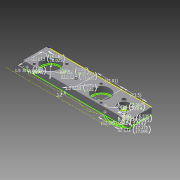
# Autodesk Inventor part: mount
Saved by Autodesk Inventor 2014 (Build 180170000, 170)
## iProperties
Created: 2013-09-13
Part Number: mount
Material: Generic
Document SubType Name: Modeling
Designer: Brandon
Density: 1 g/cm^3
Appearance: Default
Author: Brandon
Autodesk Inventor part; units mm, degrees
ref_plane "YZ Plane" through (0, 0, 0) normal (1, 0, 0) x (0, 1, 0)
ref_plane "XZ Plane" through (0, 0, 0) normal (0, 1, 0) x (-1, 0, 0)
ref_plane "XY Plane" through (0, 0, 0) normal (0, 0, 1) x (1, 0, 0)
sketch "Sketch1" plane through (0, 0, 0) normal (0, 0, 1) x (1, 0, 0)
  circle A0 centre (0, 0) radius 0.88
  circle A1 centre (-15.0103, 0) radius 6.031
  line L0 (0, 7.7873) -> (0, -6.2127)
  line L1 (-25, -6.2127) -> (37, -6.2127)
  line L2 (-25, 7.7873) -> (-25, -6.2127)
  circle A2 centre (-15.0103, 0) radius 5.1925
  line L3 (-15.0103, 0) -> (-8.4, 0) construction
  line L4 (-15.0103, 0) -> (-8.4, 0) construction
  circle A3 centre (-10.1801, 4.8302) radius 0.775
  circle A4 centre (-19.8406, -4.8302) radius 0.75
  circle A5 centre (15.0103, 0) radius 6.031
  circle A6 centre (15.0103, 0) radius 5.1925
  line L5 (15.0103, 0) -> (8.4, 0) construction
  line L6 (15.0103, 0) -> (8.4, 0) construction
  circle A7 centre (10.1801, 4.8302) radius 0.775
  circle A8 centre (19.8406, -4.8302) radius 0.75
  line L7 (15.0103, 0) -> (-15.0103, 0)
  circle A9 centre (28.5103, -0.0028) radius 4.5042 construction
  circle A10 centre (28.5103, -0.0028) radius 8.6375
  line L8 (28.5103, -0.0028) -> (32.1014, -0.0028) construction
  circle A11 centre (24.9041, 3.6034) radius 1.132
  circle A12 centre (32.1166, -3.609) radius 1.132
  line L9 (0, -6.2127) -> (0.0002, -7.8127) construction
  line L10 (0.0002, -7.8127) -> (-19.9998, -7.815) construction
  line L11 (0.0002, -7.8127) -> (20.0002, -7.8104) construction
  circle A13 centre (15.0103, 0) radius 8.9958 construction
  circle A14 centre (28.5103, -0.0028) radius 2.5 construction
  circle A15 centre (28.5103, -0.0028) radius 3.2675
  line L12 (15.0103, 0) -> (28.5103, -0.0028)
  line L13 (32.1166, -3.609) -> (24.9041, 3.6034) construction
  line L14 (35.2985, -0.4271) -> (28.086, 6.7854)
  line L15 (21.7221, 0.4215) -> (28.9346, -6.791)
  arc A16 (28.9346, -6.791) -> (35.2985, -0.4271) centre (32.1166, -3.609) ccw
  arc A17 (28.086, 6.7854) -> (21.7221, 0.4215) centre (24.9041, 3.6034) ccw
  circle A18 centre (28.5103, -0.0028) radius 7.7
  circle A19 centre (28.5103, -0.0028) radius 3.5
  line L16 (-25, 7.7873) -> (37, 7.7873)
  line L17 (37, 7.7873) -> (37, -6.2127)
  line L18 (22.5067, -6.2127) -> (34.5139, -6.2127) construction
  line L19 (0.0002, -7.8127) -> (-0.0008, -11.0127) construction
  line L20 (-0.0008, -11.0127) -> (29.997, -11.0219) construction
  line L21 (-0.0008, -11.0127) -> (-30.0008, -11.0035) construction
  line L22 (-0.0008, -11.0127) -> (29.9992, -11.0127) construction
  circle A20 centre (0, 0) radius 6 construction
  line L23 (-15.0103, 0) -> (-10.7457, 4.2646) construction
  line L24 (-15.0103, 0) -> (-19.2749, -4.2646) construction
  line L25 (-10.7457, 4.2646) -> (-10.1801, 4.8302) construction
  line L26 (-19.2749, -4.2646) -> (-19.8406, -4.8302) construction
  line L27 (-19.2749, -4.2646) -> (-18.4749, -4.2646) construction
  dimension "d0" = 1.5
  dimension "d3" = 11.6
  dimension "d8" = 10
  dimension "d13" = 1.5
  dimension "d14" = 1.5
  dimension "d26" = 17
  dimension "d31" = 2
  dimension "d32" = 2
  dimension "d38" = 5
  dimension "d40" = 6.15
  dimension "d42" = 15.0103
  dimension "d52" = 13.5
  dimension "d53" = 9
  dimension "d54" = 7
  dimension "d60" = 12.0072
  dimension "d81" = 1.6
  dimension "d86" = 3.2
  dimension "d87" = 45
  dimension "d88" = 10.2
  dimension "d89" = 12
  dimension "d90" = 0.8
  dimension "d91" = 0.8
  dimension "d92" = 135
  dimension "d98" = 14
  constraints: 58 end point, 21 centre point, 12 coincident, 8 point on circle, 7 horizontal, 6 collinear, 6 symmetric about line, 5 tangent, 4 perpendicular, 4 point on line, 2 equal length, 1 midpoint, 1 parallel, 4 other
  measures "d14" diameter of A4
  measures "d38" diameter of A14
  measures "d42" distance of point (0, 0) A5.centre
  measures "d52" distance of L12.start L8.start
  measures "d53" diameter of A17
  measures "d54" diameter of A19
  measures "d60" distance of L18.start L18.end
  measures "d81" distance of L9.end L0.end
  measures "d86" distance of L9.end L19.end
  measures "d87" angle of L8 L13
  measures "d88" distance of L13.start L13.end
  measures "d89" diameter of A20
  measures "d90" distance of L23.end L25.end
  measures "d91" distance of L24.end L26.end
  measures "d92" angle of L26 L27
  measures "d98" distance of L2.start L1.start
extrude "Extrusion5" add sketch "Sketch1" along normal blind 4 contours L7 L0 A0 | L7 A5 A10 L1 L0 A0 | A0 L0 L16 A17 A10 A5 L7 | A0 L0 L7 | L0 L7 A0 | A0 L0 L1 L2 L16 | A0 L7 L0 | L7 A6 A10 A5 | A5 A10 A6 L7 | A10 A17 A5 | A5 A18 L12 A6 A10 | A10 A6 L12 A18 A5 | A5 A18 L1 A10 | L16 A10 A17 | A17 A18 A5 | A17 A10 L16 A18 | A18 L12 A5 | A5 L12 L15 L1 A18 | A18 A17 L15 L12 A5 | A5 L12 A18 | A18 A17 L14 A16 L1 L15 | L16 L17 A10 | A10 L17 A16 A18 A17 L16 | A10 A16 L1 | L1 A18 A16 A10 | A16 A10 L17 L1 | A18 A16 L14 A17 | A1 picked at (22.6351, 6.7046) picked at (35.2187, -5.8987) picked at (34.0103, -5.7745)
extrude "Extrusion6" add sketch "Sketch1" along normal blind 0.6 contours A19
extrude "Extrusion7" add sketch "Sketch1" against normal blind 1 contours A18 L12 A5 | A5 L12 L15 L1 A18 | L1 L15 A16 A18 | A18 A17 L15 L12 A5 | A5 L12 A18 | A18 A17 L14 A16 L1 L15 | L1 A18 A16 L15 | A18 A16 L14 A17 | A19
extrude "Extrusion8" add sketch "Sketch1" against normal blind 2 contours L16 A10 A17 | A17 A10 L16 | A17 A10 L16 A18 | A17 L16 A10 | A16 A18 L1 A10 | A10 L1 A16 | A18 A17 L14 A16 L1 L15 | L1 A18 A16 L15 | A10 A16 L1 | L1 A18 A16 A10 | A19 picked at (22.6351, 6.7046) picked at (23.9954, 7.8592) picked at (25.8454, 7.8295) picked at (33.7332, -6.4634) picked at (31.1737, -6.4131) picked at (34.0103, -5.7745)
extrude "Extrusion9" cut sketch "Sketch1" against normal up to surface (1 mm away) from surface at -1 contours A10 A17 A5 | A5 A18 L12 A6 A10 | A10 A6 L12 A18 A5 | A5 A18 L1 A10 | A17 A18 A5 | A17 A10 L16 A18 | A6 L12 A10 | A18 L12 A5 | A5 L12 L15 L1 A18 | A10 L12 A6 | A17 L16 A10 | A10 L16 A17 | A18 A17 L15 L12 A5 | A5 L12 A18 | A18 A17 L14 A16 L1 L15 | A10 L17 A16 A18 A17 L16 | L1 A18 A16 A10 | A18 A16 L14 A17 | A10 L17 | A19 picked at (25.8454, 7.8295) picked at (29.8002, 7.9844) picked at (34.0103, -5.7745)
extrude "Extrusion10" cut sketch "Sketch1" against normal blind 2 contours L7 L0 A0 | L7 A5 A10 L1 L0 A0 | A0 L0 L16 A17 A10 A5 L7 | A0 L0 L7 | A10 A17 A5 | A5 A18 L1 A10 | L16 A10 A17 | A17 A18 A5 | A17 A10 L16 A18 | A5 L12 L15 L1 A18 | A18 A17 L15 L12 A5 | A18 A17 L14 A16 L1 L15 | L16 L17 A10 | A10 L17 A16 A18 A17 L16 | A10 A16 L1 | L1 A18 A16 A10 | A16 A10 L17 L1 | A18 A16 L14 A17 keep common part picked at (0.4122, 0.4122) picked at (0.4122, -0.4122) picked at (22.6351, 6.7046) picked at (35.2187, -5.8987) picked at (34.0103, -5.7745)
extrude "Extrusion11" add sketch "Sketch1" along normal blind 4 contours L7 L0 A0 | L7 A5 A10 L1 L0 A0 | A0 L0 L16 A17 A10 A5 L7 | A0 L0 L7 | L0 L7 A0 | A0 L0 L1 L2 L16 | A0 L7 L0 | L7 A6 A10 A5 | A5 A10 A6 L7 | A10 A17 A5 | A5 A18 L12 A6 A10 | A10 A6 L12 A18 A5 | A5 A18 L1 A10 | L16 A10 A17 | A17 A18 A5 | A17 A10 L16 A18 | A18 L12 A5 | A5 L12 L15 L1 A18 | A18 A17 L15 L12 A5 | A5 L12 A18 | A18 A17 L14 A16 L1 L15 | L16 L17 A10 | A10 L17 A16 A18 A17 L16 | A10 A16 L1 | L1 A18 A16 A10 | A16 A10 L17 L1 | A18 A16 L14 A17 | A1 picked at (22.6351, 6.7046) picked at (35.2187, -5.8987) picked at (34.0103, -5.7745)
extrude "Extrusion12" add sketch "Sketch1" against normal blind 1 contours A19
extrude "Extrusion13" add sketch "Sketch1" along normal blind 0.5 contours A19
extrude "Extrusion14" cut sketch "Sketch1" along normal blind 0.9 contours L7 A6 A10 A5 | A5 A10 A6 L7 | A5 A18 L12 A6 A10 | A10 A6 L12 A18 A5 | A18 L12 A5 | A5 L12 A18 | A1
extrude "Extrusion15" cut sketch "Sketch1" along normal blind 10 contours L7 L0 A0 | A0 L0 L7 | L0 L7 A0 | A0 L7 L0
sketch "Sketch2" plane through (24.7792, 7.7873, -1) normal (0, 1, 0) x (1, 0, 0)
  line L0 (12.2208, -5) -> (-49.7792, -5) projected
  line L1 (-49.7792, -5) -> (-48.1994, -5)
  line L2 (-45.7792, -1) -> (-49.7792, -1)
  line L3 (-49.7792, -1) -> (-49.7792, -5)
  circle A0 centre (-47.7792, -3) radius 1.25
  line L4 (-24.7792, -1) -> (-24.7792, -5)
  circle A1 centre (-1.7792, -3) radius 1.25
  dimension "d95" = 4
  dimension "d97" = 2.5
  constraints: 8 end point, 2 centre point, 2 point on line, 1 horizontal, 1 parallel, 1 perpendicular, 1 symmetric about line, 1 other
  measures "d95" distance of L2.end L2.start
  measures "d97" diameter of A0
extrude "Extrusion16" cut sketch "Sketch2" against normal blind 14 contours A0
extrude "Extrusion17" cut sketch "Sketch2" against normal blind 14 contours A1
body "Solid3"
